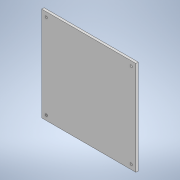
# Autodesk Inventor part: hank - base 1
Saved by Autodesk Inventor 2022 (Build 260153000, 153)
## iProperties
Created: 2021-01-16
Part Number: hank - base 1
Material: Generic
Document SubType Name: Modeling
Designer: chris
Density: 1 g/cm^3
Appearance: Default
Author: chris
Autodesk Inventor part; units mm, degrees
ref_plane "YZ Plane" through (0, 0, 0) normal (1, 0, 0) x (0, 1, 0)
ref_plane "XZ Plane" through (0, 0, 0) normal (0, 1, 0) x (-1, 0, 0)
ref_plane "XY Plane" through (0, 0, 0) normal (0, 0, 1) x (1, 0, 0)
sketch "Sketch1" plane through (0, 0, 0) normal (0, 0, 1) x (1, 0, 0)
  line L0 (-63.5, 63.5) -> (63.5, 63.5)
  line L1 (63.5, 63.5) -> (63.5, -63.5)
  line L2 (63.5, -63.5) -> (-63.5, -63.5)
  line L3 (-63.5, -63.5) -> (-63.5, 63.5)
  circle A0 centre (-57.15, 57.15) radius 1.524
  circle A1 centre (57.15, 57.15) radius 1.524
  line L4 (63.5, 0) -> (-63.5, 0)
  circle A2 centre (-57.15, -57.15) radius 1.524
  circle A3 centre (57.15, -57.15) radius 1.524
  point P0 (0, 0)
  point P1 (0, 63.5)
  dimension "d0" = 127
  dimension "d1" = 127
  dimension "d2" = 127
  dimension "d3" = 3.048
  dimension "d4" = 3.048
  dimension "d5" = 6.35
  dimension "d6" = 6.35
  dimension "d7" = 6.35
  dimension "d8" = 6.35
  constraints: 10 end point, 4 centre point, 3 midpoint, 2 perpendicular, 2 symmetric about line, 1 horizontal, 1 horizontal alignment, 1 vertical alignment, 2 other
  measures "d0" distance of L0.start L0.end
  measures "d1" distance of L0.end L1.end
  measures "d2" distance of L1.end L2.end
  measures "d3" diameter of A0
  measures "d4" diameter of A1
  measures "d5" distance from line of L3 A0.centre
  measures "d6" distance from line of L0 A0.centre
  measures "d7" distance from line of L0 A1.centre
  measures "d8" distance from line of L1 A1.centre
extrude "Extrusion1" add sketch "Sketch1" along normal blind 3.175
body "Solid1"
